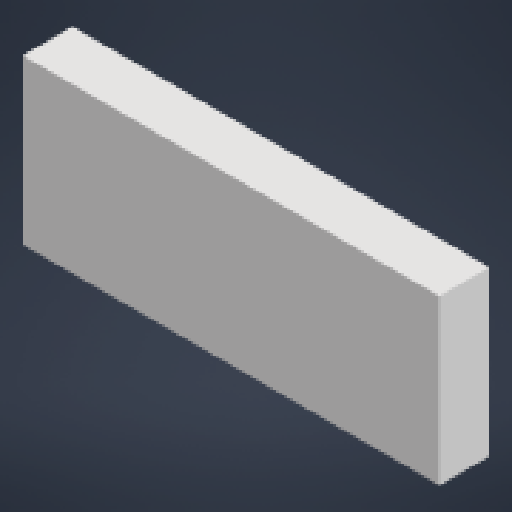
# Autodesk Inventor part: Part5
Saved by Autodesk Inventor 2025.2 (Build 292293000, 293)
## iProperties
Created: 2025-03-05
Part Number: Part5
Material: Generic
Document SubType Name: Modeling
Designer: cbast
Density: 1 g/cm^3
Appearance: Default
Author: cbast
Autodesk Inventor part; units mm, degrees
ref_plane "YZ Plane" through (0, 0, 0) normal (1, 0, 0) x (0, 1, 0)
ref_plane "XZ Plane" through (0, 0, 0) normal (0, 1, 0) x (-1, 0, 0)
ref_plane "XY Plane" through (0, 0, 0) normal (0, 0, 1) x (1, 0, 0)
sketch "Sketch1" plane through (0, 0, 0) normal (0, 0, 1) x (1, 0, 0)
  line L0 (166.6929, -8) -> (166.6929, 6) projected
  line L1 (0, 6) -> (166.6929, 6) projected
  line L2 (0, -8) -> (0, 6) projected
  line L3 (166.6929, -8) -> (0, -8) projected
  line L4 (0, -45.5) -> (0, -59.5) projected
  line L5 (166.6929, -59.5) -> (0, -59.5) projected
  line L6 (166.6929, -45.5) -> (166.6929, -59.5) projected
  line L7 (0, -45.5) -> (166.6929, -45.5) projected
  line L8 (0, 6) -> (166.6929, 6)
  line L9 (166.6929, 6) -> (166.6929, -59.5)
  line L10 (166.6929, -59.5) -> (0, -59.5)
  line L11 (0, -59.5) -> (0, 6)
  point P0 (0, 0)
  constraints: 8 end point, 2 parallel, 1 horizontal, 1 perpendicular
extrude "Extrusion1" add sketch "Sketch1" along normal blind 20
body "Solid1"
